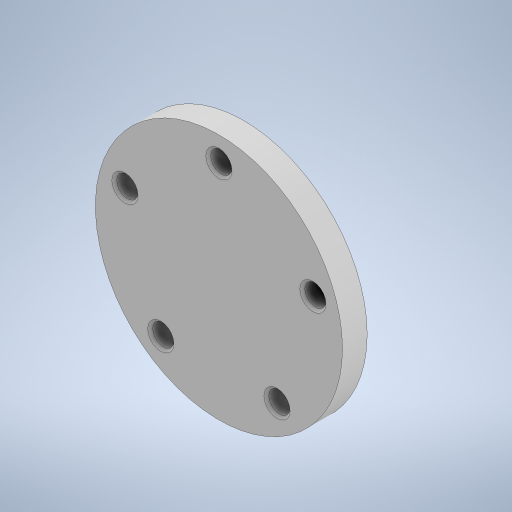
# Autodesk Inventor part: 회전축 상단
Saved by Autodesk Inventor 2023 (Build 270158000, 158)
## iProperties
Created: 2022-06-21
Part Number: 회전축 상단
Material: 일반
Document SubType Name: Modeling
Designer: user
Density: 1 g/cm^3
Appearance: 기본값
Author: user
Autodesk Inventor part; units mm, degrees
ref_plane "YZ Plane" through (0, 0, 0) normal (1, 0, 0) x (0, 1, 0)
ref_plane "XZ Plane" through (0, 0, 0) normal (0, 1, 0) x (-1, 0, 0)
ref_plane "XY Plane" through (0, 0, 0) normal (0, 0, 1) x (1, 0, 0)
sketch "스케치1" plane through (0, 0, 0) normal (0, 0, 1) x (1, 0, 0)
  circle A0 centre (0, 0) radius 20 construction
  circle A1 centre (0, 20) radius 2.15
  circle A2 centre (-19.0211, 6.1803) radius 2.15
  circle A3 centre (-11.7557, -16.1803) radius 2.15
  circle A4 centre (11.7557, -16.1803) radius 2.15
  circle A5 centre (19.0211, 6.1803) radius 2.15
  circle A6 centre (0, 0) radius 25
  dimension "d0" = 40
  dimension "d1" = 4.3
  dimension "d4" = 360
  dimension "d6" = 50
  constraints: 6 centre point, 2 coincident, 1 vertical alignment, 13 other
  measures "d1" diameter of A1
  measures "d6" diameter of A6
extrude "돌출1" add sketch "스케치1" along normal blind 5
sketch "스케치2" plane through (0, 0, 0) normal (0, 0, -1) x (-1, 0, 0)
  circle A0 centre (0, 0) radius 7.35
  dimension "d9" = 14.7
  constraints: 1 centre point, 1 coincident
  measures "d9" diameter of A0
extrude "돌출2" add sketch "스케치2" along normal blind 10
chamfer "모따기1" distance 0.5 angle 45 5 edges at (-21.1711, 6.1803, 5) (-2.15, 20, 5) (16.8711, 6.1803, 5) (9.6057, -16.1803, 5) (-13.9057, -16.1803, 5)
sketch "스케치3" plane through (0, 0, -10) normal (0, 0, -1) x (-1, 0, 0)
  circle A0 centre (0, 0) radius 7.35 projected
  line L0 (4, 6.1662) -> (4, -6.1662)
  dimension "d15" = 4
  constraints: 2 end point, 2 point on circle, 1 vertical
  measures "d15" distance from line of point (0, 0) L0
extrude "돌출3" cut sketch "스케치3" against normal blind 10 contours A0 L0 picked at (5.1167, 0)
